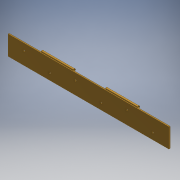
# Autodesk Inventor part: Hinge 1 of 2
Saved by Autodesk Inventor 2018 (Build 220112000, 112)
## iProperties
Created: 2018-10-30
Part Number: Hinge 1 of 2
Material: Brass, Soft Yellow
Document SubType Name: Modeling
Designer: P301319
Density: 8.47 g/cm^3
Appearance: Brass - Satin
Author: P301319
Autodesk Inventor part; units mm, degrees
ref_plane "YZ Plane" through (0, 0, 0) normal (1, 0, 0) x (0, 1, 0)
ref_plane "XZ Plane" through (0, 0, 0) normal (0, 1, 0) x (-1, 0, 0)
ref_plane "XY Plane" through (0, 0, 0) normal (0, 0, 1) x (1, 0, 0)
sketch "Sketch1" plane through (0, 0, 0) normal (0, 1, 0) x (-1, 0, 0)
  line L0 (0, 0) -> (-250, 0)
  line L1 (-250, 0) -> (-250, -30)
  line L2 (-250, -30) -> (0, -30)
  line L3 (0, -30) -> (0, 0)
  dimension "d0" = 250
  dimension "d1" = 30
  constraints: 8 end point, 2 parallel, 1 horizontal, 1 perpendicular
  measures "d0" distance of L2.end L1.end
  measures "d1" distance of L1.end L0.end
extrude "Extrusion1" add sketch "Sketch1" along normal blind 2
sketch "Sketch2" plane through (250, 0, 0) normal (1, 0, 0) x (0, 0, -1)
  circle A0 centre (0, 3) radius 1.25
  circle A1 centre (0, 3) radius 1.75
  point P0 (0, 0)
  dimension "d4" = 2.5
  dimension "d5" = 3
  dimension "d6" = 3.5
  constraints: 2 centre point, 1 coincident, 1 vertical alignment
  measures "d4" diameter of A0
  measures "d5" distance of point (0, 0) A0.centre
  measures "d6" diameter of A1
extrude "Extrusion2" add sketch "Sketch2" against normal blind 250
extrude "Extrusion3" cut sketch "Sketch2" against normal blind 250 contours A0
sketch "Sketch3" plane through (250, 0, -30) normal (0, 0, -1) x (-1, 0, 0)
  line L0 (0, 2) -> (250, 2) projected
  line L1 (0, 2) -> (50, 2)
  line L2 (50, 2) -> (50, 4.75)
  line L3 (50, 4.75) -> (0, 4.75)
  line L4 (0, 4.75) -> (0, 2)
  line L5 (100, 4.75) -> (150, 4.75)
  line L6 (150, 4.75) -> (150, 2)
  line L7 (150, 2) -> (100, 2)
  line L8 (100, 2) -> (100, 4.75)
  line L9 (200, 4.75) -> (250, 4.75)
  line L10 (250, 4.75) -> (250, 2)
  line L11 (250, 2) -> (200, 2)
  line L12 (200, 2) -> (200, 4.75)
  point P0 (250, 0)
  point P1 (125, 2)
  point P2 (125, 2)
  point P3 (225, 2)
  dimension "d11" = 50
  dimension "d12" = 2.75
  dimension "d13" = 50
  dimension "d14" = 2.75
  dimension "d15" = 50
  dimension "d16" = 50
  dimension "d17" = 2.75
  dimension "d18" = 50
  constraints: 24 end point, 6 parallel, 3 horizontal, 3 midpoint, 3 perpendicular, 1 coincident, 1 horizontal alignment
  measures "d11" distance of L3.end L2.end
  measures "d12" distance of L2.end L1.end
  measures "d13" distance of L6.end L7.end
  measures "d14" distance of L5.end L6.end
  measures "d15" distance between parallel lines of L2 L8
  measures "d16" distance of L10.end L11.end
  measures "d17" distance of L9.end L10.end
  measures "d18" distance between parallel lines of L6 L12
extrude "Extrusion4" cut sketch "Sketch3" against normal through all
sketch "Sketch4" plane through (200, 2, 1.4361) normal (0, 1, 0) x (1, 0, 0)
  line L0 (-200, 1.4361) -> (-200, 0) projected
  line L1 (-150, 0) -> (-200, 0) projected
  line L2 (-200, 1.4361) -> (-150, 1.4361)
  line L3 (-150, 1.4361) -> (-150, 0)
  line L4 (-150, 0) -> (-200, 0)
  line L5 (-200, 0) -> (-200, 1.4361)
  line L6 (-100, 0.1861) -> (-100, 2.6861) projected
  line L7 (-50, 0.6861) -> (-50, 0) projected
  line L8 (-100, 1.4361) -> (-50, 1.4361)
  line L9 (-50, 1.4361) -> (-50, 0)
  line L10 (-50, 0) -> (-100, 0)
  line L11 (-100, 0) -> (-100, 1.4361)
  line L12 (50, 2.1861) -> (50, 0.6861) projected
  line L13 (50, 0) -> (0, 0) projected
  line L14 (50, 1.4361) -> (0, 1.4361)
  line L15 (0, 1.4361) -> (0, 0)
  line L16 (0, 0) -> (50, 0)
  line L17 (50, 0) -> (50, 1.4361)
  point P0 (-100, 2.1861)
  point P1 (-100, 0.6861)
  constraints: 24 end point, 6 parallel, 3 horizontal, 3 perpendicular, 2 midpoint
extrude "Extrusion5" cut sketch "Sketch4" against normal through all
sketch "Sketch5" plane through (0, 2, 0) normal (0, 1, 0) x (1, 0, 0)
  line L0 (100, 1.75) -> (100, -1.75) projected
  line L1 (0, 0) -> (50, 0) projected
  point P0 (25, 10)
  point P1 (65, 20)
  point P2 (105, 10)
  point P3 (145, 20)
  point P4 (185, 10)
  point P5 (225, 20)
  point P6 (100, 0)
  point P7 (100, 1.4361)
  dimension "d23" = 40
  dimension "d24" = 5
  dimension "d25" = 40
  dimension "d26" = 40
  dimension "d27" = 40
  dimension "d28" = 40
  dimension "d29" = 10
  dimension "d30" = 10
  constraints: 4 horizontal alignment
  measures "d23" horizontal distance of point (145, 20) point (105, 10)
  measures "d24" distance from line of point (105, 10) L0
  measures "d25" horizontal distance of point (105, 10) point (65, 20)
  measures "d26" horizontal distance of point (65, 20) point (25, 10)
  measures "d27" horizontal distance of point (145, 20) point (185, 10)
  measures "d28" horizontal distance of point (185, 10) point (225, 20)
  measures "d29" vertical distance of point (25, 10) point (65, 20)
  measures "d30" distance from line of L1 point (25, 10)
hole "Hole1" at (25, 2, -10) at (65, 2, -20) at (105, 2, -10) at (145, 2, -20) at (185, 2, -10) at (225, 2, -20) direction (0, -1, 0) diameter 3 end through all countersink diameter 5 countersink angle 90
equation "\"d13\" = d11"
equation "\"d15\" = d11"
equation "\"d16\" = d11"
equation "\"d18\" = d11"
equation "\"d25\" = d23"
equation "\"d26\" = d23"
equation "\"d27\" = d23"
equation "\"d28\" = d23"
body "Solid1"
